Filament Swatch (Autodesk Fusion 360 design; units mm, degrees)
Autodesk Fusion 360 part; units mm, degrees
sketch "Sketch1" plane through (0, 0, 0) normal (0, 0, 1) x (1, 0, 0)
  line L0 (0, 0) -> (40, 0)
  line L1 (40, 0) -> (40, 30)
  line L2 (40, 30) -> (0, 30)
  line L3 (0, 30) -> (0, 0)
  line L4 (0, 12) -> (40, 12)
  line L5 (8, 12) -> (8, 0)
  line L6 (14.4, 12) -> (14.4, 0)
  line L7 (20.8, 12) -> (20.8, 0)
  line L8 (27.2, 12) -> (27.2, 0)
  line L9 (33.6, 12) -> (33.6, 0)
  circle A0 centre (4, 4) radius 2.5
  line L10 (2.5, 27.5) -> (37.5, 27.5)
  line L11 (37.5, 27.5) -> (37.5, 14.5)
  line L12 (37.5, 14.5) -> (2.5, 14.5)
  line L13 (2.5, 14.5) -> (2.5, 27.5)
  line L14 (8, 4) -> (0, 4) construction
  dimension "d3" = 6.4
  dimension "d4" = 6.4
  dimension "d5" = 6.4
  dimension "d6" = 6.4
  dimension "d9" = 40
  dimension "d24" = 5
  dimension "d29" = 13
  dimension "d32" = 30
  dimension "d33" = 2.5
  dimension "d34" = 2.5
  dimension "d35" = 2.5
  dimension "d39" = 2.5
  dimension "d42" = 12
  dimension "d43" = 35
  dimension "d44" = 4
  dimension "d45" = 8
  constraint horizontal L0
  constraint vertical L1
  constraint horizontal L2
  constraint vertical L3
  constraint coincident L0.start L3.end
  constraint coincident L3 L4.start
  constraint coincident L1 L4.end
  constraint perpendicular L1 L4
  constraint coincident L4 L5.start
  constraint coincident L0 L5.end
  constraint perpendicular L0 L5
  constraint coincident L4 L6.start
  constraint coincident L0 L6.end
  constraint perpendicular L0 L6
  constraint coincident L4 L7.start
  constraint coincident L0 L7.end
  constraint perpendicular L0 L7
  constraint coincident L4 L8.start
  constraint coincident L0 L8.end
  constraint perpendicular L0 L8
  constraint coincident L4 L9.start
  constraint coincident L0 L9.end
  constraint perpendicular L0 L9
  constraint horizontal L10
  constraint vertical L11
  constraint horizontal L12
  constraint vertical L13
  constraint coincident L5 L14.start
  constraint coincident L3 L14.end
  constraint perpendicular L3 L14
  constraint midpoint A0.centre L14
  measures "d3" distance of L5 L6
  measures "d4" distance of L6 L7
  measures "d5" distance of L7 L8
  measures "d6" distance of L8 L9
  measures "d9" distance of L1.end L2.end
  measures "d24" diameter of A0
  measures "d29" distance of L10.start L12.end
  measures "d32" distance of L0 L2
  measures "d33" distance of L2 L10
  measures "d34" distance of L4 L12
  measures "d35" distance of L1 L11
  measures "d39" distance of L3 L13
  measures "d42" distance of L9.start L9.end
  measures "d43" distance of L10.start L10.end
  measures "d44" distance of L0 A0.centre
  measures "d45" distance of L3 L5
extrude "Extrude1" add sketch "Sketch1" along normal blind 1.2 contours L0 L3 L4 L5 | L1 L2 L3 L4 | A0 | L10 L11 L12 L13 makes body 1
extrude "Extrude2" add sketch "Sketch1" along normal blind 0.2 contours L0 L4 L5 L6 bodies 1
extrude "Extrude3" add sketch "Sketch1" along normal blind 0.4 contours L0 L4 L6 L7 bodies 1
extrude "Extrude4" add sketch "Sketch1" along normal blind 0.6 contours L0 L4 L7 L8 bodies 1
extrude "Extrude5" add sketch "Sketch1" along normal blind 0.8 contours L0 L4 L8 L9 bodies 1
extrude "Extrude6" add sketch "Sketch1" along normal blind 1 contours L0 L1 L4 L9 bodies 1
extrude "Extrude7" cut sketch "Sketch1" along normal up to surface (1.2 mm away) contours A0 bodies 1
extrude "Extrude8" cut sketch "Sketch1" against normal blind 0.4 from surface at 1.2 contours L10 L11 L12 L13 bodies 1
fillet "Fillet1" radius 3 4 edges at (0, 0, 0.6) (0, 30, 0.6) (40, 30, 0.6) (40, 0, 0.5) on bodies 1
sketch "Sketch1 (2)" plane through (0, 0, 0) normal (0, 0, 1) x (1, 0, 0) in component "Flexible swatch "
  line L0 (93.5349, 4.5302) -> (128.5349, 4.5302)
  line L1 (128.5349, 4.5302) -> (128.5349, -8.4698)
  line L2 (128.5349, -8.4698) -> (93.5349, -8.4698)
  line L3 (93.5349, -8.4698) -> (93.5349, 4.5302)
  line L4 (111.0349, 4.5302) -> (111.0349, -8.4698) construction
  line L5 (86.0349, 23.0302) -> (136.0349, 23.0302)
  line L6 (136.0349, 23.0302) -> (136.0349, -26.9698)
  line L7 (136.0349, -26.9698) -> (86.0349, -26.9698)
  line L8 (86.0349, -26.9698) -> (86.0349, 23.0302)
  line L9 (86.0349, 23.0302) -> (136.0349, -26.9698) construction
  line L10 (136.0349, 23.0302) -> (86.0349, -26.9698) construction
  circle A0 centre (99.2099, 9.8552) radius 3.175
  line L11 (96.0349, 9.8552) -> (96.0349, 15.7856) construction
  point P0 (111.0349, -1.9698)
  dimension "d46" = 13
  dimension "d47" = 35
  dimension "d48" = 50
  dimension "d49" = 50
  dimension "d56" = 6.35
  dimension "d59" = 13.175
  dimension "d60" = 13.175
  constraint horizontal L0
  constraint vertical L1
  constraint horizontal L2
  constraint vertical L3
  constraint midpoint L0 L4.start
  constraint midpoint L2 L4.end
  constraint horizontal L5
  constraint perpendicular L5 L6
  constraint parallel L5 L7
  constraint parallel L6 L8
  constraint coincident L9 P0
  constraint coincident L10 P0
  constraint midpoint L4 P0
  constraint coincident A0 L11.start
  constraint parallel L8 L11
  constraint tangent A0 L11
  measures "d46" distance of L0.start L2.end
  measures "d47" distance of L0.start L0.end
  measures "d48" distance of L5.start L7.end
  measures "d49" distance of L5.start L5.end
  measures "d56" diameter of A0
  measures "d59" distance of L8 A0.centre
  measures "d60" distance of L5 A0.centre
extrude "Extrude1'" add sketch "Sketch1 (2)" along normal blind 1.6 separate body makes body 2 in component "Flexible swatch "
fillet "Fillet1'" radius 6 4 edges at (86.0349, -26.9698, 0.8) (86.0349, 23.0302, 0.8) (136.0349, -26.9698, 0.8) (136.0349, 23.0302, 0.8) on bodies 2 in component "Flexible swatch "
extrude "Extrude2'" add sketch "Sketch1 (2)" along normal blind 1.4 contours L0 L1 L2 L3 bodies 2 in component "Flexible swatch "
component "Flexible swatch " placed x (1, 0, 0) y (0, 1, 0) z (0, 0, 1) at (0, 0, 0)
equation "d3 = ( d9 - d45 ) / 5"
equation "d4 = d3"
equation "d5 = d3"
equation "d6 = d3"
equation "d49 = d48"
equation "d59 = 10 mm + ( 0.5 * d56 )"
equation "d60 = d59"
named bodies: "Filament Swatch", "Flexible Material Secondary Swatch"
